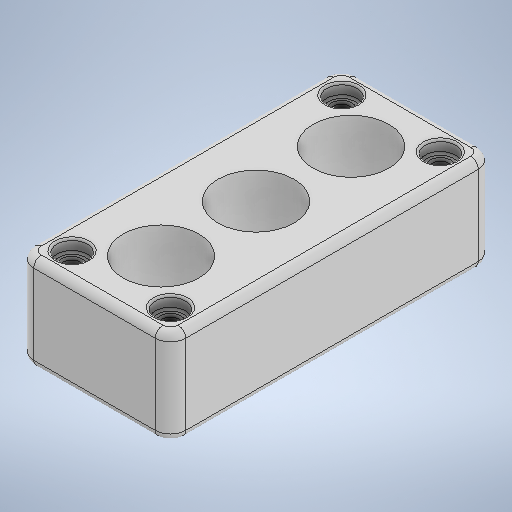
# Autodesk Inventor part: guia superior
Saved by Autodesk Inventor 2025.2 (Build 292293000, 293)
## iProperties
Created: 2025-10-16
Part Number: guia superior
Material: Genérico
Document SubType Name: Modeling
Designer: Jonathan Galarza
Density: 1 g/cm^3
Appearance: Valor por defecto
Author: Jonathan Galarza
Autodesk Inventor part; units mm, degrees
ref_plane "YZ Plane" through (0, 0, 0) normal (1, 0, 0) x (0, 1, 0)
ref_plane "XZ Plane" through (0, 0, 0) normal (0, 1, 0) x (-1, 0, 0)
ref_plane "XY Plane" through (0, 0, 0) normal (0, 0, 1) x (1, 0, 0)
sketch "Boceto1" plane through (0, 0, 0) normal (0, 1, 0) x (-1, 0, 0)
  line L0 (-20, -42.5) -> (20, -42.5)
  line L1 (20, -42.5) -> (20, 42.5)
  line L2 (20, 42.5) -> (-20, 42.5)
  line L3 (-20, 42.5) -> (-20, -42.5)
  line L4 (-20, -42.5) -> (20, 42.5) construction
  line L5 (20, -42.5) -> (-20, 42.5) construction
  line L6 (15.6711, 0) -> (-15.6711, 0) construction
  line L7 (0, 25) -> (0, -25) construction
  circle A0 centre (0, 25) radius 7.5
  circle A1 centre (0, -25) radius 7.5
  circle A2 centre (0, 25) radius 10
  circle A3 centre (0, -25) radius 10
  circle A4 centre (0, 0) radius 10
  circle A5 centre (-13, -35.5) radius 2.25
  line L8 (15.6711, 0) -> (-15.6711, 0)
  line L9 (0, -12.7103) -> (0, 13.5129)
  circle A6 centre (-13, 35.5) radius 2.25
  circle A7 centre (13, -35.5) radius 2.25
  circle A8 centre (13, 35.5) radius 2.25
  point P0 (0, 35)
  point P1 (0, -35)
  dimension "d0" = 40
  dimension "d1" = 85
  dimension "d3" = 50
  dimension "d6" = 15
  dimension "d7" = 15
  dimension "d8" = 20
  dimension "d27" = 4.5
  dimension "d28" = 7
  dimension "d29" = 7
  constraints: 20 end point, 9 centre point, 5 coincident, 4 midpoint, 3 horizontal, 3 symmetric about line, 2 parallel, 2 point on line, 1 perpendicular, 1 vertical, 3 other
  measures "d0" distance of L2.end L1.end
  measures "d1" distance of L1.end L0.end
  measures "d3" distance of L7.start L7.end
  measures "d6" diameter of A0
  measures "d7" diameter of A1
  measures "d8" diameter of A4
  measures "d27" diameter of A5
  measures "d28" distance from line of L3 A5.centre
  measures "d29" distance from line of L0 A5.centre
extrude "Extrusión1" add sketch "Boceto1" along normal blind 25 contours L3 L2 L1 L0
fillet "Empalme1" radius 4 4 edges at (20, 12.5, -42.5) (20, 12.5, 42.5) (-20, 12.5, 42.5) (-20, 12.5, -42.5)
fillet "Empalme2" radius 2 16 edges at (-18.8284, 25, 41.3284) (0, 25, 42.5) (18.8284, 25, 41.3284) (20, 25, 0) (18.8284, 25, -41.3284) (0, 25, -42.5) (-18.8284, 25, -41.3284) (-20, 25, 0) (-18.8284, 0, 41.3284) (0, 0, 42.5) (18.8284, 0, 41.3284) (20, 0, 0) (18.8284, 0, -41.3284) (0, 0, -42.5) (-18.8284, 0, -41.3284) (-20, 0, 0)
sketch "Boceto3" plane through (0, 25, 0) normal (0, 1, 0) x (1, 0, 0)
  circle A0 centre (13, 35.5) radius 2.25 projected
  circle A1 centre (13, 35.5) radius 4
  line L0 (-7.5192, 0) -> (7.6222, 0)
  line L1 (0.0515, -5.5954) -> (0.0515, 7.1321)
  circle A2 centre (13, -35.5) radius 4
  circle A3 centre (-12.897, 35.5) radius 4
  circle A4 centre (-12.897, -35.5) radius 4
  point P0 (0, 0)
  dimension "d30" = 8
  constraints: 4 centre point, 4 end point, 3 symmetric about line, 1 coincident, 1 horizontal, 1 vertical, 3 other
  measures "d30" diameter of A1
extrude "Extrusión4" cut sketch "Boceto3" against normal blind 3.25 contours A0 | A1 | A2 | A3 | A4
fillet "Empalme3" radius 0.5 4 edges at (-16.897, 25, 35.5) (9, 25, 35.5) (9, 25, -35.5) (-16.897, 25, -35.5)
fillet "Empalme4" radius 0.5 12 edges at (-16.897, 21.75, -35.5) (-10.75, 21.75, -35.5) (9, 21.75, -35.5) (15.25, 21.75, -35.5) (-10.75, 21.75, 35.5) (-16.897, 21.75, 35.5) (9, 21.75, 35.5) (15.25, 21.75, 35.5) (15.25, 0, 35.5) (-10.75, 0, 35.5) (15.25, 0, -35.5) (-10.75, 0, -35.5)
